Autodesk Fusion 360 part; units mm, degrees
(part 3 of 4)
  measures "d44" distance of L104.start L104.end
  measures "d45" distance of L104.start L106.end
  measures "d46" distance of L108.start L108.end
  measures "d47" distance of L108.start L110.end
  measures "d48" distance of L112.start L112.end
  measures "d49" distance of L112.start L114.end
  measures "d50" distance of L116.start L116.end
  measures "d51" distance of L116.start L118.end
  measures "d52" distance of L120.start L120.end
  measures "d53" distance of L120.start L122.end
  measures "d54" distance of L124.start L124.end
  measures "d55" distance of L124.start L126.end
  measures "d56" distance of L128.start L128.end
  measures "d57" distance of L128.start L130.end
  measures "d58" distance of L132.start L132.end
  measures "d59" distance of L132.start L134.end
  measures "d60" distance of L136.start L136.end
  measures "d61" distance of L136.start L138.end
  measures "d62" distance of L140.start L140.end
  measures "d63" distance of L140.start L142.end
  measures "d64" distance of L144.start L144.end
  measures "d65" distance of L144.start L146.end
  measures "d66" distance of L18.end L148.end
  measures "d67" distance of L18.end L150.end
  measures "d68" distance of L26.end L152.end
  measures "d69" distance of L26.end L154.end
  measures "d70" distance of L34.end L156.end
  measures "d71" distance of L34.end L158.end
  measures "d72" distance of L160.start L160.end
  measures "d73" distance of L160.start L162.end
  measures "d74" distance of L164.start L164.end
  measures "d75" distance of L164.start L166.end
  measures "d76" distance of L168.start L168.end
  measures "d77" distance of L168.start L170.end
  measures "d78" distance of L172.start L172.end
  measures "d79" distance of L172.start L174.end
  measures "d80" distance of L176.start L176.end
  measures "d81" distance of L176.start L178.end
  measures "d82" distance of L180.start L180.end
  measures "d83" distance of L180.start L182.end
  measures "d84" distance of L184.start L184.end
  measures "d85" distance of L184.start L186.end
  measures "d86" distance of L188.start L188.end
  measures "d87" distance of L188.start L190.end
  measures "d88" distance of L192.start L192.end
  measures "d89" distance of L192.start L194.end
  measures "d90" distance of L196.start L196.end
  measures "d91" distance of L196.start L198.end
  measures "d92" distance of L200.start L200.end
  measures "d93" distance of L200.start L202.end
  measures "d94" distance of L86.end L204.end
  measures "d95" distance of L86.end L206.end
  measures "d96" distance of L94.end L208.end
  measures "d97" distance of L94.end L210.end
  measures "d98" distance of L212.start L212.end
  measures "d99" distance of L212.start L214.end
  measures "d100" distance of L78.end L216.end
  measures "d101" distance of L78.end L218.end
  measures "d102" distance of L70.end L220.end
  measures "d103" distance of L70.end L222.end
  measures "d104" distance of L42.end L224.end
  measures "d105" distance of L42.end L226.end
  measures "d106" distance of L50.end L228.end
  measures "d107" distance of L50.end L230.end
  measures "d108" distance of L58.end L232.end
  measures "d109" distance of L58.end L234.end
  measures "d110" distance of L0.end L236.end
  measures "d111" distance of L0.end L238.end
  measures "d112" diameter of A0
  measures "d113" diameter of A1
  measures "d114" diameter of A2
  measures "d115" diameter of A3
  measures "d116" diameter of A4
  measures "d117" diameter of A5
  measures "d118" diameter of A6
  measures "d119" diameter of A7
  measures "d120" diameter of A8
  measures "d121" diameter of A9
  measures "d122" diameter of A10
  measures "d123" diameter of A11
  measures "d124" diameter of A12
  measures "d125" diameter of A13
  measures "d126" diameter of A14
  measures "d127" diameter of A15
  measures "d128" diameter of A16
  measures "d129" diameter of A17
  measures "d130" diameter of A18
  measures "d131" diameter of A19
  measures "d132" diameter of A20
  measures "d133" diameter of A21
  measures "d134" diameter of A22
  measures "d135" diameter of A23
  measures "d136" diameter of A24
  measures "d137" diameter of A25
  measures "d138" diameter of A26
  measures "d139" diameter of A27
  measures "d140" diameter of A28
  measures "d141" diameter of A29
  measures "d142" diameter of A30
  measures "d143" diameter of A31
  measures "d144" diameter of A32
  measures "d146" diameter of A33
  measures "d149" distance of L12 A21.centre
  measures "d150" distance of A21.centre A23.centre
  measures "d151" distance of P2 A23.centre
  measures "d152" distance of P3 P2
  measures "d154" distance of L148 A0.centre
  measures "d155" distance of L7 A21.centre
  measures "d156" distance of A21.centre A22.centre
  measures "d157" distance of A22.centre A25.centre
  measures "d158" distance of A25.centre A27.centre
  measures "d159" distance of A27.centre A29.centre
  measures "d160" distance of A29.centre A31.centre
  measures "d164" distance of A32.centre A33.centre
  measures "d167" distance of A14.centre A15.centre
  measures "d168" distance of L240.start L240.end
  measures "d169" distance of L241.start L241.end
  measures "d170" distance of A10.centre A17.centre
  measures "d171" distance of L0 A0.centre
  measures "d172" horizontal distance of L238.end A6.centre
  measures "d173" distance of L95 A7.centre
  measures "d174" distance of L87 A14.centre
  measures "d175" distance of L79 A33.centre
  measures "d177" diameter of A34
extrude "Extrude4" cut sketch "Sketch3" against normal blind 50 contours L217 A33 L247 | L217 A33 L247 | L205 A14 L247 | L205 A14 L247 | L209 A7 L247 | L209 A7 L247 | A21 L242 | A21 L242 | A23 L242 L243 | A23 L242 L243 | A23 L242 L243 | A23 L242 L243 | A20 L242 L244 | A20 L242 L244 | A20 L242 L244 | A20 L242 L244 | A13 L242 L245 | A13 L242 L245 | A13 L242 L245 | A13 L242 L245 | A0 L240 L246 | A0 L240 L242 | A0 L240 L242 L246 | L154 A1 L246 | L154 A1 L246 | L158 A2 L246 | L158 A2 L246 | L201 A15 | L201 A15 | L226 A3 L246 | L226 A3 L246 | L230 A4 L246 | L230 A4 L246 | L234 A5 L246 | L234 A5 L246 | L237 A6 L246 | L237 L238 A6 L246 | L238 A6 L246 L247 | A6 L246 L247 | A8 | A9 | A10 | A11 | A12 | A16 | A17 | A18 | A19 | A22 | A24 | A25 | A26 | A27 | A28 | A29 | A30 | A31 | A32
extrude "Extrude3" cut sketch "Sketch3" against normal blind 50 contours L221 L247 A34 | L221 L247 A34 | L217 A33 L247 | L217 A33 L247 | L205 A14 L247 | L205 A14 L247 | L209 A7 L247 | L209 A7 L247 | A21 L242 | A21 L242 | A23 L242 L243 | A23 L242 L243 | A23 L242 L243 | A23 L242 L243 | A20 L242 L244 | A20 L242 L244 | A20 L242 L244 | A20 L242 L244 | A13 L242 L245 | A13 L242 L245 | A13 L242 L245 | A13 L242 L245 | A0 L240 L246 | A0 L240 L242 | A0 L240 L242 L246 | L154 A1 L246 | L154 A1 L246 | L158 A2 L246 | L158 A2 L246 | L201 A15 | L201 A15 | L226 A3 L246 | L226 A3 L246 | L230 A4 L246 | L230 A4 L246 | L234 A5 L246 | L234 A5 L246 | L237 A6 L246 | L237 L238 A6 L246 | L238 A6 L246 L247 | A6 L246 L247 | A8 | A9 | A10 | A11 | A12 | A16 | A17 | A18 | A19 | A22 | A24 | A25 | A26 | A27 | A28 | A29 | A30 | A31 | A32

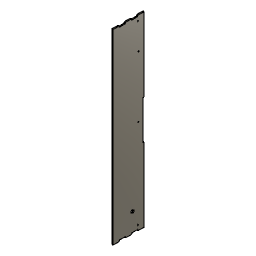
design "C2. Bordes Laterales.Salida fuente.v3"
Autodesk Fusion 360 part; units mm, degrees
ref_plane "WorkPlane1" through (0, 3, 0) normal (0, 1, 0) x (0, 0, 1)
sketch "Sketch1" plane through (0, 3, 0) normal (0, 1, 0) x (1, 0, 0)
  line L0 (340.5, 241.5) -> (-340.5, 241.5) construction
  line L1 (-340.5, 241.5) -> (-340.5, -241.5) construction
  line L2 (-340.5, -241.5) -> (340.5, -241.5) construction
  line L3 (340.5, -241.5) -> (340.5, 241.5) construction
  line L4 (340.5, 241.5) -> (-340.5, -241.5) construction
  line L5 (-340.5, 241.5) -> (340.5, -241.5) construction
  line L6 (-340.5, 241.5) -> (-337.5, 241.5)
  line L7 (-337.5, 241.5) -> (-337.5, -241.5)
  line L8 (-337.5, -241.5) -> (-340.5, -241.5)
  line L9 (-340.5, -241.5) -> (-340.5, 241.5)
  dimension "d2" = 681
  dimension "d3" = 483
  dimension "d4" = 3
  constraint horizontal L0
  constraint perpendicular L0 L1
  constraint parallel L0 L2
  constraint parallel L1 L3
  constraint coincident L4 origin
  constraint coincident L5 origin
  constraint horizontal L6
  constraint vertical L7
  constraint horizontal L8
  constraint vertical L9
  measures "d2" distance of L1.end L2.end
  measures "d3" distance of L0.end L1.end
  measures "d4" distance of L0.end L6.end
extrude "Extrude1" add sketch "Sketch1" along normal blind 80
ref_plane "WorkPlane2" through (-340.5, 43, 0) normal (-1, 0, 0) x (0, 0, 1)
sketch "Sketch2" plane through (-340.5, 42, 0) normal (-1, 0, 0) x (0, 1, 0)
  line L0 (-39, 241.5) -> (-39, -241.5)
  line L1 (-39, -241.5) -> (41, -241.5)
  line L2 (41, -241.5) -> (41, 241.5)
  line L3 (41, 241.5) -> (-39, 241.5)
  line L4 (0, 0) -> (0, -50) construction
  line L5 (0, 0) -> (0, 50) construction
  line L6 (41, 50) -> (38, 50)
  line L7 (38, 50) -> (38, -50)
  line L8 (38, -50) -> (41, -50)
  line L9 (41, -50) -> (41, 50)
  line L10 (-39, 241.5) -> (-23, 241.5)
  line L11 (-23, 241.5) -> (-23, 244.5)
  line L12 (-23, 244.5) -> (-39, 244.5)
  line L13 (-39, 244.5) -> (-39, 241.5)
  line L14 (-23, 241.5) -> (-7, 241.5)
  line L15 (-7, 241.5) -> (-7, 238.5)
  line L16 (-7, 238.5) -> (-23, 238.5)
  line L17 (-23, 238.5) -> (-23, 241.5)
  line L18 (-7, 241.5) -> (9, 241.5)
  line L19 (9, 241.5) -> (9, 244.5)
  line L20 (9, 244.5) -> (-7, 244.5)
  line L21 (-7, 244.5) -> (-7, 241.5)
  line L22 (9, 241.5) -> (25, 241.5)
  line L23 (25, 241.5) -> (25, 238.5)
  line L24 (25, 238.5) -> (9, 238.5)
  line L25 (9, 238.5) -> (9, 241.5)
  line L26 (-39, -241.5) -> (-23, -241.5)
  line L27 (-23, -241.5) -> (-23, -244.5)
  line L28 (-23, -244.5) -> (-39, -244.5)
  line L29 (-39, -244.5) -> (-39, -241.5)
  line L30 (-23, -241.5) -> (-7, -241.5)
  line L31 (-7, -241.5) -> (-7, -238.5)
  line L32 (-7, -238.5) -> (-23, -238.5)
  line L33 (-23, -238.5) -> (-23, -241.5)
  line L34 (-7, -241.5) -> (9, -241.5)
  line L35 (9, -241.5) -> (9, -244.5)
  line L36 (9, -244.5) -> (-7, -244.5)
  line L37 (-7, -244.5) -> (-7, -241.5)
  line L38 (9, -241.5) -> (25, -241.5)
  line L39 (25, -241.5) -> (25, -238.5)
  line L40 (25, -238.5) -> (9, -238.5)
  line L41 (9, -238.5) -> (9, -241.5)
  line L42 (25, -241.5) -> (40, -241.5)
  line L43 (25, -241.5) -> (41, -241.5)
  line L44 (41, -241.5) -> (41, -244.5)
  line L45 (41, -244.5) -> (25, -244.5)
  line L46 (25, -244.5) -> (25, -241.5)
  line L47 (25, 241.5) -> (41, 241.5)
  line L48 (41, 241.5) -> (41, 244.5)
  line L49 (41, 244.5) -> (25, 244.5)
  line L50 (25, 244.5) -> (25, 241.5)
  dimension "d8" = 50
  dimension "d9" = 50
  dimension "d10" = 3
  dimension "d11" = 16
  dimension "d12" = 3
  dimension "d13" = 16
  dimension "d14" = 3
  dimension "d15" = 16
  dimension "d16" = 3
  dimension "d17" = 16
  dimension "d18" = 3
  dimension "d20" = 16
  dimension "d21" = 3
  dimension "d22" = 16
  dimension "d23" = 3
  dimension "d24" = 16
  dimension "d25" = 3
  dimension "d26" = 16
  dimension "d27" = 3
  dimension "d31" = 3
  dimension "d32" = 3
  constraint coincident L4.start L5.start
  constraint parallel L0 L4
  constraint vertical L5
  constraint horizontal L6
  constraint vertical L7
  constraint horizontal L8
  constraint vertical L9
  constraint coincident L2 L6.start
  constraint horizontal L10
  constraint vertical L11
  constraint horizontal L12
  constraint vertical L13
  constraint coincident L0.start L3.end
  constraint horizontal L14
  constraint vertical L15
  constraint horizontal L16
  constraint vertical L17
  constraint horizontal L18
  constraint vertical L19
  constraint horizontal L20
  constraint vertical L21
  constraint horizontal L22
  constraint vertical L23
  constraint horizontal L24
  constraint vertical L25
  constraint horizontal L26
  constraint vertical L27
  constraint horizontal L28
  constraint vertical L29
  constraint coincident L0.end L1.start
  constraint horizontal L30
  constraint vertical L31
  constraint horizontal L32
  constraint vertical L33
  constraint horizontal L34
  constraint vertical L35
  constraint horizontal L36
  constraint vertical L37
  constraint horizontal L38
  constraint vertical L39
  constraint horizontal L40
  constraint vertical L41
  constraint horizontal L42
  constraint horizontal L43
  constraint vertical L44
  constraint horizontal L45
  constraint vertical L46
  constraint horizontal L47
  constraint vertical L48
  constraint horizontal L49
  constraint vertical L50
  measures "d8" distance of L4.start L4.end
  measures "d9" distance of L4.start L5.end
  measures "d10" distance of L6.start L6.end
  measures "d11" distance of L0.start L10.end
  measures "d12" distance of L0.start L12.end
  measures "d13" distance of L10.end L14.end
  measures "d14" distance of L10.end L16.end
  measures "d15" distance of L14.end L18.end
  measures "d16" distance of L14.end L20.end
  measures "d17" distance of L18.end L22.end
  measures "d18" distance of L18.end L24.end
  measures "d20" distance of L0.end L26.end
  measures "d21" distance of L0.end L28.end
  measures "d22" distance of L26.end L30.end
  measures "d23" distance of L26.end L32.end
  measures "d24" distance of L30.end L34.end
  measures "d25" distance of L30.end L36.end
  measures "d26" distance of L34.end L38.end
  measures "d27" distance of L34.end L40.end
  measures "d31" distance of L38.end L45.end
  measures "d32" distance of L22.end L49.end
extrude "Extrude2" cut sketch "Sketch2" against normal blind 25 contours L3 L14 L15 L16 L17 | L1 L30 L31 L32 L33 | L3 L22 L23 L24 L25 | L1 L38 L39 L40 L41 | L2 L6 L7 L8 L9
ref_plane "WorkPlane3" through (-337.5, 43, 0) normal (1, 0, 0) x (0, 0, -1)
sketch "Sketch3" plane through (-337.5, 43, 0) normal (1, 0, 0) x (0, 1, 0)
  line L0 (37, 50) -> (40, 50)
  line L1 (40, 50) -> (40, 241.5)
  line L2 (40, 241.5) -> (24, 241.5)
  line L3 (24, 241.5) -> (24, 238.5)
  line L4 (24, 238.5) -> (8, 238.5)
  line L5 (8, 238.5) -> (8, 241.5)
  line L6 (8, 241.5) -> (-8, 241.5)
  line L7 (-8, 241.5) -> (-8, 238.5)
  line L8 (-8, 238.5) -> (-24, 238.5)
  line L9 (-24, 238.5) -> (-24, 241.5)
  line L10 (-24, 241.5) -> (-40, 241.5)
  line L11 (-40, 241.5) -> (-40, -241.5)
  line L12 (-40, -241.5) -> (-24, -241.5)
  line L13 (-24, -241.5) -> (-24, -238.5)
  line L14 (-24, -238.5) -> (-8, -238.5)
  line L15 (-8, -238.5) -> (-8, -241.5)
  line L16 (-8, -241.5) -> (8, -241.5)
  line L17 (8, -241.5) -> (8, -238.5)
  line L18 (8, -238.5) -> (24, -238.5)
  line L19 (24, -238.5) -> (24, -241.5)
  line L20 (24, -241.5) -> (40, -241.5)
  line L21 (40, -241.5) -> (40, -50)
  line L22 (40, -50) -> (37, -50)
  line L23 (37, -50) -> (37, 50)
ref_plane "WorkPlane4" through (-337.5, 43, 0) normal (1, 0, 0) x (0, 0, -1)
sketch "Sketch4" plane through (-337.5, 43, 0) normal (1, 0, 0) x (0, 1, 0)
  line L0 (37, -50) -> (37, 50)
  line L1 (37, 10) -> (19, 10)
  line L2 (19, 10) -> (19, -10)
  line L3 (19, -10) -> (37, -10)
  line L4 (37, -10) -> (37, 10)
  line L5 (37, 10) -> (19, -10) construction
  line L6 (19, 10) -> (37, -10) construction
  circle A0 centre (25, 2) radius 1.5
  circle A1 centre (10, -191.5) radius 4
  line L7 (37, 50) -> (37, 260) construction
  circle A2 centre (24, 228.5) radius 1.5
  line L8 (19, 238.5) -> (19, 218.5)
  line L9 (19, 218.5) -> (37, 218.5)
  line L10 (37, 218.5) -> (37, 238.5)
  line L11 (37, 238.5) -> (19, 238.5)
  line L12 (0, 0) -> (6.2879, 0)
  circle A3 centre (24, -228.5) radius 1.5
  line L13 (19, -218.5) -> (37, -218.5)
  line L14 (37, -218.5) -> (37, -238.5)
  line L15 (37, -238.5) -> (19, -238.5)
  line L16 (19, -238.5) -> (19, -218.5)
  line L17 (40, 241.5) -> (45, 241.5)
  line L18 (45, 241.5) -> (45, 141.5)
  line L19 (37, 161.5) -> (19, 161.5)
  line L20 (19, 161.5) -> (19, 141.5)
  line L21 (19, 141.5) -> (37, 141.5)
  line L22 (37, 141.5) -> (37, 161.5)
  circle A4 centre (26, 159.346) radius 1.5
  line L23 (37, 238.5) -> (42, 238.5)
  line L24 (42, 238.5) -> (42, 161.5)
  line L25 (40, 241.5) -> (40, 50)
  line L26 (24, 241.5) -> (40, 241.5)
  line L27 (28, 241.5) -> (28, 228.5)
  line L28 (24, -241.5) -> (40, -241.5)
  line L29 (40, -50) -> (40, -241.5)
  line L30 (87.333, 241.5) -> (87.333, 159.346)
  line L31 (87.333, 159.346) -> (-5, 159.346)
  point P0 (-0.5, -125.5)
  point P1 (28, 0)
  point P2 (37, 238.5)
  point P3 (37, -238.5)
  point P4 (40, 241.5)
  point P5 (26, 159.346)
  dimension "d47" = 20
  dimension "d53" = 3
  dimension "d54" = 18
  dimension "d61" = 8
  dimension "d64" = 3
  dimension "d65" = 18
  dimension "d66" = 100
  dimension "d67" = 3
  dimension "d68" = 18
  dimension "d69" = 77
  dimension "d70" = 13
  dimension "d71" = 16
  dimension "d72" = 13
  dimension "d73" = 12
  dimension "d74" = 14
  dimension "d75" = 12
  dimension "d76" = 16
  dimension "d77" = 82.154
  dimension "d78" = 82.154
  constraint horizontal L1
  constraint perpendicular L1 L2
  constraint parallel L1 L3
  constraint parallel L2 L4
  constraint coincident L5 P1
  constraint coincident L6 P1
  constraint horizontal L11
  constraint vertical L8
  constraint horizontal L9
  constraint vertical L10
  constraint coincident L12.start origin
  constraint horizontal L12
  constraint symmetric P2 L12 P3
  constraint symmetric L8.end L12 L13.start
  constraint symmetric L8.start L12 L15.end
  constraint symmetric L9.end L12 L13.end
  constraint symmetric A2 L12 A3
  constraint coincident P4 L17.start
  constraint perpendicular L7 L17
  constraint perpendicular L11 L18
  constraint horizontal L19
  constraint vertical L20
  constraint horizontal L21
  constraint vertical L22
  constraint coincident P2 L10.end
  constraint perpendicular L10 L23
  constraint perpendicular L19 L24
  constraint coincident L26 L27.start
  constraint perpendicular L26 L27
  constraint perpendicular L17 L30
  constraint perpendicular L22 L31
  constraint coincident L31 P5
  measures "d47" distance of L1.end L2.end
  measures "d53" diameter of A0
  measures "d54" distance of L1.start L1.end
  measures "d61" diameter of A1
  measures "d64" diameter of A2
  measures "d65" distance of P2 L8.start
  measures "d66" distance of L17.end L18.end
  measures "d67" diameter of A4
  measures "d68" distance of L19.end L19.start
  measures "d69" distance of L23.end L24.end
  measures "d70" distance of L27.start L27.end
  measures "d71" distance of A3.centre L29
  measures "d72" distance of A3.centre L28
  measures "d73" distance of L4 A0.centre
  measures "d74" distance of P5 L25
  measures "d75" distance of L25 L27.end
  measures "d76" distance of A2.centre L25
  measures "d77" distance of L30.start L30.end
  measures "d78" distance of L30.start L30.end
extrude "Extrude3" cut sketch "Sketch4" against normal blind 20 contours A0 | A1 | A2 | A3 | A4 L31 | A4 L31

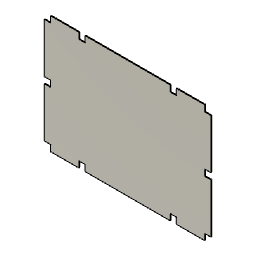
design "D.Pantalla cartnegro.v3"
Autodesk Fusion 360 part; units mm, degrees
ref_plane "WorkPlane1" through (0, 22, 0) normal (0, 1, 0) x (0, 0, 1)
sketch "Sketch1" plane through (0, 22, 0) normal (0, 1, 0) x (1, 0, 0)
  line L0 (337.5, -238.5) -> (-337.5, -238.5)
  line L1 (-337.5, -238.5) -> (-337.5, 238.5)
  line L2 (-337.5, 238.5) -> (337.5, 238.5)
  line L3 (337.5, 238.5) -> (337.5, -238.5)
  line L4 (337.5, -238.5) -> (-337.5, 238.5) construction
  line L5 (-337.5, -238.5) -> (337.5, 238.5) construction
  dimension "d2" = 675
  dimension "d3" = 477
  constraint horizontal L0
  constraint perpendicular L0 L1
  constraint parallel L0 L2
  constraint parallel L1 L3
  constraint coincident L4 origin
  constraint coincident L5 origin
  measures "d2" distance of L1.end L2.end
  measures "d3" distance of L0.end L1.end
extrude "Extrude1" add sketch "Sketch1" along normal blind 3
ref_plane "WorkPlane2" through (0, 22, 0) normal (0, -1, 0) x (-1, 0, 0)
sketch "Sketch2" plane through (0, 22, 0) normal (0, -1, 0) x (1, 0, 0)
  line L0 (-337.5, -238.5) -> (337.5, -238.5)
  line L1 (337.5, -238.5) -> (337.5, 238.5)
  line L2 (337.5, 238.5) -> (-337.5, 238.5)
  line L3 (-337.5, 238.5) -> (-337.5, -238.5)
  line L4 (337.5, 238.5) -> (312.5, 238.5)
  line L5 (312.5, 238.5) -> (312.5, 213.5)
  line L6 (312.5, 213.5) -> (337.5, 213.5)
  line L7 (337.5, 213.5) -> (337.5, 238.5)
  line L8 (-337.5, 238.5) -> (-312.5, 238.5)
  line L9 (-312.5, 238.5) -> (-312.5, 213.5)
  line L10 (-312.5, 213.5) -> (-337.5, 213.5)
  line L11 (-337.5, 213.5) -> (-337.5, 238.5)
  line L12 (-337.5, -238.5) -> (-312.5, -238.5)
  line L13 (-312.5, -238.5) -> (-312.5, -213.5)
  line L14 (-312.5, -213.5) -> (-337.5, -213.5)
  line L15 (-337.5, -213.5) -> (-337.5, -238.5)
  line L16 (337.5, -238.5) -> (312.5, -238.5)
  line L17 (312.5, -238.5) -> (312.5, -213.5)
  line L18 (312.5, -213.5) -> (337.5, -213.5)
  line L19 (337.5, -213.5) -> (337.5, -238.5)
  line L20 (337.5, 12.5) -> (312.5, 12.5)
  line L21 (312.5, 12.5) -> (312.5, -12.5)
  line L22 (312.5, -12.5) -> (337.5, -12.5)
  line L23 (337.5, -12.5) -> (337.5, 12.5)
  line L24 (337.5, 12.5) -> (312.5, -12.5) construction
  line L25 (312.5, 12.5) -> (337.5, -12.5) construction
  line L26 (-337.5, 12.5) -> (-337.5, -12.5)
  line L27 (-312.5, -12.5) -> (-312.5, 12.5)
  line L28 (-312.5, -238.5) -> (-312.5, 238.5)
  line L29 (-337.5, -12.5) -> (-312.5, -12.5)
  line L30 (-337.5, 12.5) -> (-312.5, -12.5) construction
  line L31 (-312.5, 12.5) -> (-337.5, -12.5) construction
  line L32 (-312.5, 12.5) -> (-337.5, 12.5)
  line L33 (-337.5, 262.49) -> (-197.5, 262.49)
  line L34 (-337.5, -260.2374) -> (-197.5, -260.2374)
  line L35 (337.5, 281.2113) -> (197.5, 281.2113)
  line L36 (-197.5, 238.5) -> (-172.5, 238.5)
  line L37 (-172.5, 238.5) -> (-172.5, 213.5)
  line L38 (-172.5, 213.5) -> (-197.5, 213.5)
  line L39 (-197.5, 213.5) -> (-197.5, 238.5)
  line L40 (197.5, 238.5) -> (172.5, 238.5)
  line L41 (172.5, 238.5) -> (172.5, 213.5)
  line L42 (172.5, 213.5) -> (197.5, 213.5)
  line L43 (197.5, 213.5) -> (197.5, 238.5)
  line L44 (337.5, -262.9157) -> (197.5, -262.9157)
  line L45 (197.5, -238.5) -> (172.5, -238.5)
  line L46 (172.5, -238.5) -> (172.5, -213.5)
  line L47 (172.5, -213.5) -> (197.5, -213.5)
  line L48 (197.5, -213.5) -> (197.5, -238.5)
  line L49 (-197.5, -238.5) -> (-172.5, -238.5)
  line L50 (-172.5, -238.5) -> (-172.5, -213.5)
  line L51 (-172.5, -213.5) -> (-197.5, -213.5)
  line L52 (-197.5, -213.5) -> (-197.5, -238.5)
  point P0 (337.5, 0)
  point P1 (325, 0)
  point P2 (-312.5, 0)
  point P3 (-325, 0)
  dimension "d7" = 25
  dimension "d8" = 25
  dimension "d9" = 25
  dimension "d10" = 25
  dimension "d11" = 25
  dimension "d12" = 25
  dimension "d13" = 25
  dimension "d14" = 25
  dimension "d17" = 140
  dimension "d18" = 140
  dimension "d19" = 140
  dimension "d20" = 25
  dimension "d21" = 25
  dimension "d22" = 25
  dimension "d23" = 25
  dimension "d24" = 140
  dimension "d25" = 25
  dimension "d26" = 25
  dimension "d27" = 25
  dimension "d28" = 25
  constraint horizontal L4
  constraint vertical L5
  constraint horizontal L6
  constraint vertical L7
  constraint coincident L1.end L2.start
  constraint horizontal L8
  constraint vertical L9
  constraint horizontal L10
  constraint vertical L11
  constraint coincident L2.end L3.start
  constraint horizontal L12
  constraint vertical L13
  constraint horizontal L14
  constraint vertical L15
  constraint coincident L0.start L3.end
  constraint horizontal L16
  constraint vertical L17
  constraint horizontal L18
  constraint vertical L19
  constraint coincident L0.end L1.start
  constraint horizontal L20
  constraint perpendicular L20 L21
  constraint parallel L20 L22
  constraint parallel L21 L23
  constraint coincident L24 P1
  constraint coincident L25 P1
  constraint horizontal L32
  constraint perpendicular L26 L32
  constraint parallel L29 L32
  constraint parallel L26 L27
  constraint coincident P3 L31
  constraint coincident P3 L30
  constraint perpendicular L3 L33
  constraint horizontal L34
  constraint perpendicular L7 L35
  constraint horizontal L36
  constraint vertical L37
  constraint horizontal L38
  constraint vertical L39
  constraint coincident L2 L36.start
  constraint horizontal L40
  constraint vertical L41
  constraint horizontal L42
  constraint vertical L43
  constraint coincident L2 L40.start
  constraint perpendicular L1 L44
  constraint horizontal L45
  constraint vertical L46
  constraint horizontal L47
  constraint vertical L48
  constraint coincident L0 L45.start
  constraint horizontal L49
  constraint vertical L50
  constraint horizontal L51
  constraint vertical L52
  constraint coincident L0 L49.start
  measures "d7" distance of L1.end L4.end
  measures "d8" distance of L1.end L6.end
  measures "d9" distance of L2.end L8.end
  measures "d10" distance of L2.end L10.end
  measures "d11" distance of L0.start L12.end
  measures "d12" distance of L0.start L14.end
  measures "d13" distance of L0.end L16.end
  measures "d14" distance of L0.end L18.end
  measures "d17" distance of L33.start L33.end
  measures "d18" distance of L34.start L34.end
  measures "d19" distance of L35.start L35.end
  measures "d20" distance of L36.start L36.end
  measures "d21" distance of L36.start L38.end
  measures "d22" distance of L40.start L40.end
  measures "d23" distance of L40.start L42.end
  measures "d24" distance of L44.start L44.end
  measures "d25" distance of L45.start L45.end
  measures "d26" distance of L45.start L47.end
  measures "d27" distance of L49.start L49.end
  measures "d28" distance of L49.start L51.end
extrude "Extrude2" cut sketch "Sketch2" against normal blind 150 contours L0 L3 L12 L13 L14 L15 L28 | L0 L49 L50 L51 L52 | L3 L26 L27 L28 L29 L32 | L0 L45 L46 L47 L48 | L2 L3 L8 L9 L10 L11 L28 | L0 L1 L16 L17 L18 L19 | L2 L36 L37 L38 L39 | L1 L20 L21 L22 L23 | L2 L40 L41 L42 L43 | L1 L2 L4 L5 L6 L7
ref_plane "WorkPlane3" through (0, 22, 0) normal (0, -1, 0) x (-1, 0, 0)
sketch "Sketch3" plane through (0, 22, 0) normal (0, -1, 0) x (1, 0, 0)
  line L0 (82.5, 1.5) -> (82.5, 16.5)
  line L1 (163.5, 16.5) -> (178.5, 16.5)
  line L2 (178.5, 241.5) -> (181.5, 241.5) construction
  circle A0 centre (171, 90) radius 1.5
  line L3 (178.5, 163.5) -> (100.5, 163.5)
  line L4 (178.5, 82.5) -> (163.5, 82.5)
  line L5 (97.5, 241.5) -> (97.5, 163.5) construction
  line L6 (181.5, 163.5) -> (181.5, 241.5) construction
  line L7 (97.5, 82.5) -> (82.5, 82.5)
  line L8 (-340.5, -82.5) -> (340.5, -82.5) construction
  line L9 (19.5, 241.5) -> (97.5, 241.5) construction
  line L10 (97.5, 241.5) -> (100.5, 241.5) construction
  line L11 (340.5, -1.5) -> (-340.5, -1.5) construction
  line L12 (82.5, 82.5) -> (82.5, 97.5)
  line L13 (97.5, 97.5) -> (97.5, 82.5)
  line L14 (340.5, 82.5) -> (340.5, 160.5)
  line L15 (259.5, 241.5) -> (259.5, 163.5) construction
  line L16 (178.5, 241.5) -> (178.5, 163.5) construction
  circle A1 centre (90, 90) radius 1.5
  line L17 (244.5, 82.5) -> (244.5, 97.5)
  line L18 (244.5, 16.5) -> (259.5, 16.5)
  line L19 (340.5, 97.5) -> (340.5, 82.5)
  circle A2 centre (171, 9) radius 1.5
  line L20 (82.5, 97.5) -> (97.5, 97.5)
  line L21 (97.5, 16.5) -> (97.5, 1.5)
  line L22 (100.5, 241.5) -> (178.5, 241.5) construction
  line L23 (340.5, 79.5) -> (340.5, 82.5)
  line L24 (340.5, 163.5) -> (262.5, 163.5)
  line L25 (100.5, 163.5) -> (100.5, 241.5) construction
  line L26 (178.5, 16.5) -> (178.5, 1.5)
  line L27 (82.5, 16.5) -> (97.5, 16.5)
  line L28 (97.5, 163.5) -> (19.5, 163.5)
  line L29 (163.5, 97.5) -> (178.5, 97.5)
  line L30 (178.5, 97.5) -> (178.5, 82.5)
  circle A3 centre (90, 9) radius 1.5
  line L31 (163.5, 82.5) -> (163.5, 97.5)
  line L32 (97.5, 1.5) -> (82.5, 1.5)
  line L33 (178.5, 1.5) -> (163.5, 1.5)
  line L34 (163.5, 1.5) -> (163.5, 16.5)
  line L35 (163.5, -64.5) -> (178.5, -64.5)
  line L36 (97.5, -79.5) -> (82.5, -79.5)
  circle A4 centre (90, -234) radius 1.5
  line L37 (97.5, -241.5) -> (82.5, -241.5)
  line L38 (340.5, 79.5) -> (-340.5, 79.5) construction
  line L39 (82.5, -79.5) -> (82.5, -64.5)
  line L40 (-340.5, -163.5) -> (340.5, -163.5) construction
  line L41 (163.5, -226.5) -> (178.5, -226.5)
  line L42 (-340.5, 82.5) -> (340.5, 82.5) construction
  line L43 (340.5, 163.5) -> (-340.5, 163.5) construction
  line L44 (97.5, -64.5) -> (97.5, -79.5)
  line L45 (82.5, -241.5) -> (82.5, -226.5)
  line L46 (163.5, -241.5) -> (163.5, -226.5)
  line L47 (163.5, -145.5) -> (178.5, -145.5)
  line L48 (-340.5, -1.5) -> (340.5, -1.5) construction
  line L49 (178.5, -226.5) -> (178.5, -241.5)
  line L50 (82.5, -64.5) -> (97.5, -64.5)
  line L51 (340.5, 241.5) -> (-340.5, 241.5) construction
  line L52 (163.5, -79.5) -> (163.5, -64.5)
  line L53 (97.5, -226.5) -> (97.5, -241.5)
  circle A5 centre (171, -153) radius 1.5
  line L54 (340.5, -1.5) -> (340.5, 1.5)
  circle A6 centre (252, 9) radius 1.5
  line L55 (325.5, 1.5) -> (325.5, 16.5)
  line L56 (97.5, -160.5) -> (82.5, -160.5)
  line L57 (259.5, 82.5) -> (244.5, 82.5)
  line L58 (340.5, 82.5) -> (325.5, 82.5)
  line L59 (340.5, -145.5) -> (340.5, -160.5)
  circle A7 centre (333, -72) radius 1.5
  line L60 (244.5, -160.5) -> (244.5, -145.5)
  line L61 (340.5, -79.5) -> (340.5, -1.5)
  line L62 (16.5, -226.5) -> (16.5, -241.5)
  line L63 (16.5, 16.5) -> (16.5, 1.5)
  circle A8 centre (252, -153) radius 1.5
  line L64 (244.5, -145.5) -> (259.5, -145.5)
  line L65 (340.5, -160.5) -> (325.5, -160.5)
  line L66 (325.5, -145.5) -> (340.5, -145.5)
  line L67 (244.5, -241.5) -> (244.5, -226.5)
  line L68 (325.5, -160.5) -> (325.5, -145.5)
  line L69 (19.5, 163.5) -> (19.5, 241.5) construction
  circle A9 centre (333, -153) radius 1.5
  line L70 (259.5, -226.5) -> (259.5, -241.5)
  line L71 (259.5, -79.5) -> (244.5, -79.5)
  line L72 (325.5, -241.5) -> (325.5, -226.5)
  line L73 (340.5, -241.5) -> (325.5, -241.5)
  line L74 (340.5, -163.5) -> (340.5, -160.5)
  line L75 (259.5, -241.5) -> (244.5, -241.5)
  line L76 (-223.5, 241.5) -> (-223.5, -241.5) construction
  line L77 (340.5, -64.5) -> (340.5, -79.5)
  line L78 (-142.5, 241.5) -> (-64.5, 241.5) construction
  line L79 (-61.5, 241.5) -> (16.5, 241.5) construction
  line L80 (-226.5, 241.5) -> (-226.5, -241.5) construction
  circle A10 centre (252, -72) radius 1.5
  line L81 (340.5, -79.5) -> (325.5, -79.5)
  line L82 (-64.5, 82.5) -> (-79.5, 82.5)
  line L83 (340.5, -82.5) -> (340.5, -79.5)
  line L84 (1.5, 82.5) -> (1.5, 97.5)
  circle A11 centre (252, -234) radius 1.5
  line L85 (16.5, -241.5) -> (16.5, 241.5) construction
  line L86 (262.5, -241.5) -> (259.5, -241.5)
  line L87 (-79.5, 16.5) -> (-64.5, 16.5)
  line L88 (244.5, -64.5) -> (259.5, -64.5)
  line L89 (-340.5, 241.5) -> (-340.5, -241.5) construction
  line L90 (178.5, -64.5) -> (178.5, -79.5)
  circle A12 centre (90, -153) radius 1.5
  line L91 (82.5, -145.5) -> (97.5, -145.5)
  line L92 (97.5, -145.5) -> (97.5, -160.5)
  circle A13 centre (171, -234) radius 1.5
  line L93 (178.5, -145.5) -> (178.5, -160.5)
  line L94 (178.5, -79.5) -> (163.5, -79.5)
  line L95 (178.5, -160.5) -> (163.5, -160.5)
  line L96 (181.5, -241.5) -> (178.5, -241.5)
  line L97 (163.5, -160.5) -> (163.5, -145.5)
  circle A14 centre (90, -72) radius 1.5
  line L98 (100.5, -241.5) -> (97.5, -241.5)
  line L99 (178.5, -241.5) -> (163.5, -241.5)
  line L100 (259.5, 97.5) -> (259.5, 82.5)
  line L101 (340.5, 1.5) -> (340.5, 79.5)
  line L102 (340.5, 160.5) -> (340.5, 163.5)
  line L103 (259.5, 163.5) -> (181.5, 163.5)
  line L104 (259.5, 1.5) -> (244.5, 1.5)
  line L105 (325.5, 82.5) -> (325.5, 97.5)
  circle A15 centre (252, 90) radius 1.5
  line L106 (262.5, 241.5) -> (340.5, 241.5) construction
  circle A16 centre (333, 90) radius 1.5
  line L107 (-340.5, 1.5) -> (340.5, 1.5) construction
  line L108 (181.5, 241.5) -> (259.5, 241.5) construction
  line L109 (259.5, 16.5) -> (259.5, 1.5)
  line L110 (340.5, 241.5) -> (340.5, 163.5) construction
  line L111 (325.5, 16.5) -> (340.5, 16.5)
  line L112 (244.5, 97.5) -> (259.5, 97.5)
  line L113 (340.5, 1.5) -> (325.5, 1.5)
  line L114 (262.5, 163.5) -> (262.5, 241.5) construction
  line L115 (325.5, 97.5) -> (340.5, 97.5)
  line L116 (340.5, 16.5) -> (340.5, 1.5)
  circle A17 centre (333, 9) radius 1.5
  line L117 (259.5, 241.5) -> (262.5, 241.5) construction
  line L118 (244.5, 1.5) -> (244.5, 16.5)
  line L119 (-340.5, -82.5) -> (-340.5, -160.5)
  line L120 (-160.5, 97.5) -> (-145.5, 97.5)
  line L121 (-145.5, 163.5) -> (-223.5, 163.5)
  line L122 (-64.5, 241.5) -> (-61.5, 241.5) construction
  line L123 (340.5, -160.5) -> (340.5, -82.5)
  circle A18 centre (9, 90) radius 1.5
  line L124 (16.5, 241.5) -> (19.5, 241.5) construction
  line L125 (-160.5, -145.5) -> (-145.5, -145.5)
  line L126 (-340.5, -1.5) -> (-340.5, -79.5)
  line L127 (16.5, 241.5) -> (16.5, 163.5) construction
  line L128 (-223.5, 241.5) -> (-145.5, 241.5) construction
  circle A19 centre (9, 9) radius 1.5
  line L129 (1.5, -160.5) -> (1.5, -145.5)
  line L130 (-340.5, 163.5) -> (-340.5, 160.5)
  line L131 (-160.5, -160.5) -> (-160.5, -145.5)
  line L132 (-79.5, 1.5) -> (-79.5, 16.5)
  line L133 (-223.5, -241.5) -> (-226.5, -241.5)
  line L134 (-145.5, -79.5) -> (-160.5, -79.5)
  line L135 (1.5, 1.5) -> (1.5, 16.5)
  line L136 (-340.5, 1.5) -> (-340.5, -1.5)
  line L137 (-145.5, -241.5) -> (-160.5, -241.5)
  line L138 (-79.5, -160.5) -> (-79.5, -145.5)
  line L139 (-64.5, 1.5) -> (-79.5, 1.5)
  line L140 (-340.5, -160.5) -> (-340.5, -163.5)
  line L141 (1.5, -79.5) -> (1.5, -64.5)
  line L142 (-79.5, 82.5) -> (-79.5, 97.5)
  line L143 (-145.5, -160.5) -> (-160.5, -160.5)
  line L144 (-64.5, 16.5) -> (-64.5, 1.5)
  line L145 (1.5, 16.5) -> (16.5, 16.5)
  line L146 (-61.5, 163.5) -> (-61.5, 241.5) construction
  circle A20 centre (-153, -234) radius 1.5
  line L147 (-142.5, -241.5) -> (-145.5, -241.5)
  circle A21 centre (-72, 9) radius 1.5
  line L148 (259.5, -64.5) -> (259.5, -79.5)
  line L149 (325.5, -64.5) -> (340.5, -64.5)
  line L150 (-160.5, -241.5) -> (-160.5, -226.5)
  line L151 (-79.5, -226.5) -> (-64.5, -226.5)
  line L152 (-64.5, -226.5) -> (-64.5, -241.5)
  line L153 (-160.5, 16.5) -> (-145.5, 16.5)
  circle A22 centre (-72, -234) radius 1.5
  line L154 (-145.5, -226.5) -> (-145.5, -241.5)
  line L155 (-64.5, 241.5) -> (-64.5, 163.5) construction
  line L156 (-160.5, -79.5) -> (-160.5, -64.5)
  line L157 (1.5, 97.5) -> (16.5, 97.5)
  line L158 (1.5, -145.5) -> (16.5, -145.5)
  line L159 (-145.5, 241.5) -> (-142.5, 241.5) construction
  line L160 (-160.5, -226.5) -> (-145.5, -226.5)
  line L161 (16.5, 82.5) -> (1.5, 82.5)
  line L162 (-145.5, -145.5) -> (-145.5, -160.5)
  line L163 (-64.5, -79.5) -> (-79.5, -79.5)
  line L164 (-145.5, 82.5) -> (-160.5, 82.5)
  circle A23 centre (-153, -72) radius 1.5
  circle A24 centre (-153, -153) radius 1.5
  line L165 (-64.5, 163.5) -> (-142.5, 163.5)
  line L166 (1.5, -241.5) -> (1.5, -226.5)
  line L167 (-64.5, 97.5) -> (-64.5, 82.5)
  line L168 (-226.5, -241.5) -> (-340.5, -241.5) construction
  circle A25 centre (9, -72) radius 1.5
  line L169 (-340.5, 79.5) -> (-340.5, 1.5)
  line L170 (16.5, 97.5) -> (16.5, 82.5)
  line L171 (-145.5, 97.5) -> (-145.5, 82.5)
  line L172 (16.5, -241.5) -> (1.5, -241.5)
  circle A26 centre (-72, 90) radius 1.5
  line L173 (16.5, -160.5) -> (1.5, -160.5)
  line L174 (-340.5, -79.5) -> (-340.5, -82.5)
  line L175 (16.5, 163.5) -> (-61.5, 163.5)
  line L176 (-145.5, 241.5) -> (-145.5, 163.5) construction
  line L177 (-340.5, 82.5) -> (-340.5, 79.5)
  line L178 (1.5, -64.5) -> (16.5, -64.5)
  circle A27 centre (9, -153) radius 1.5
  line L179 (-223.5, 163.5) -> (-223.5, 241.5) construction
  circle A28 centre (-72, -72) radius 1.5
  line L180 (-340.5, 241.5) -> (-226.5, 241.5) construction
  line L181 (-64.5, -241.5) -> (-79.5, -241.5)
  line L182 (-160.5, -64.5) -> (-145.5, -64.5)
  line L183 (-64.5, -145.5) -> (-64.5, -160.5)
  line L184 (-79.5, -145.5) -> (-64.5, -145.5)
  circle A29 centre (-72, -153) radius 1.5
  line L185 (-226.5, 241.5) -> (-223.5, 241.5) construction
  line L186 (-79.5, 97.5) -> (-64.5, 97.5)
  line L187 (16.5, -79.5) -> (1.5, -79.5)
  line L188 (19.5, -241.5) -> (16.5, -241.5)
  line L189 (-340.5, 160.5) -> (-340.5, 82.5)
  line L190 (-160.5, 82.5) -> (-160.5, 97.5)
  line L191 (-142.5, 163.5) -> (-142.5, 241.5) construction
  line L192 (-64.5, -64.5) -> (-64.5, -79.5)
  line L193 (16.5, 1.5) -> (1.5, 1.5)
  line L194 (-145.5, 16.5) -> (-145.5, 1.5)
  line L195 (-79.5, -64.5) -> (-64.5, -64.5)
  line L196 (16.5, -145.5) -> (16.5, -160.5)
  line L197 (-64.5, -160.5) -> (-79.5, -160.5)
  line L198 (-79.5, -241.5) -> (-79.5, -226.5)
  line L199 (-145.5, 1.5) -> (-160.5, 1.5)
  circle A30 centre (-153, 90) radius 1.5
  line L200 (-160.5, 1.5) -> (-160.5, 16.5)
  line L201 (1.5, -226.5) -> (16.5, -226.5)
  line L202 (-145.5, -64.5) -> (-145.5, -79.5)
  line L203 (-79.5, -79.5) -> (-79.5, -64.5)
  line L204 (16.5, -64.5) -> (16.5, -79.5)
  line L205 (-61.5, -241.5) -> (-64.5, -241.5)
  circle A31 centre (-153, 9) radius 1.5
  circle A32 centre (9, -234) radius 1.5
  line L206 (-340.5, -79.5) -> (340.5, -79.5) construction
  line L207 (259.5, -241.5) -> (259.5, 241.5) construction
  line L208 (-340.5, 160.5) -> (340.5, 160.5) construction
  line L209 (340.5, 82.5) -> (-340.5, 82.5) construction
  line L210 (-340.5, -241.5) -> (-340.5, 241.5) construction
  line L211 (181.5, 241.5) -> (181.5, -241.5) construction
  circle A33 centre (171, -72) radius 1.5
  line L212 (262.5, 241.5) -> (262.5, -241.5) construction
  line L213 (340.5, -79.5) -> (-340.5, -79.5) construction
  line L214 (82.5, -160.5) -> (82.5, -145.5)
  line L215 (340.5, -82.5) -> (-340.5, -82.5) construction
  line L216 (-145.5, -241.5) -> (-145.5, 241.5) construction
  line L217 (340.5, 160.5) -> (-340.5, 160.5) construction
  line L218 (340.5, 1.5) -> (-340.5, 1.5) construction
  line L219 (340.5, -241.5) -> (340.5, 241.5) construction
  line L220 (325.5, -226.5) -> (340.5, -226.5)
  line L221 (325.5, -79.5) -> (325.5, -64.5)
  line L222 (259.5, -160.5) -> (244.5, -160.5)
  line L223 (-340.5, -241.5) -> (340.5, -241.5) construction
  line L224 (340.5, -226.5) -> (340.5, -241.5)
  line L225 (-226.5, -241.5) -> (-226.5, 241.5) construction
  circle A34 centre (333, -234) radius 1.5
  line L226 (-340.5, 79.5) -> (340.5, 79.5) construction
  line L227 (82.5, -226.5) -> (97.5, -226.5)
  line L228 (100.5, 241.5) -> (100.5, -241.5) construction
  line L229 (97.5, -241.5) -> (97.5, 241.5) construction
  line L230 (19.5, 241.5) -> (19.5, -241.5) construction
  line L231 (-340.5, -160.5) -> (340.5, -160.5) construction
  line L232 (340.5, -160.5) -> (-340.5, -160.5) construction
  line L233 (-142.5, 241.5) -> (-142.5, -241.5) construction
  line L234 (244.5, -79.5) -> (244.5, -64.5)
  line L235 (-64.5, -241.5) -> (-64.5, 241.5) construction
  line L236 (259.5, -145.5) -> (259.5, -160.5)
  line L237 (178.5, -241.5) -> (178.5, 241.5) construction
  line L238 (-61.5, 241.5) -> (-61.5, -241.5) construction
  line L239 (-172.5, -238.5) -> (-172.5, -228.5)
  circle A35 centre (-153, -228.4307) radius 1.5
  line L240 (-172.5, -228.5) -> (-154.5, -228.436)
  circle A36 centre (-72, -228.1428) radius 1.5
  line L241 (-151.5, -228.4254) -> (-73.5, -228.1481)
  circle A37 centre (9, -227.8549) radius 1.5
  line L242 (-70.5, -228.1375) -> (7.5, -227.8602)
  circle A38 centre (90, -227.567) radius 1.5
  line L243 (10.5, -227.8495) -> (88.5, -227.5723)
  circle A39 centre (171, -227.2791) radius 1.5
  circle A40 centre (252, -226.9912) radius 1.5
  line L244 (244.5, -226.5) -> (250.5827, -226.5)
  line L245 (253.4173, -226.5) -> (259.5, -226.5)
  line L246 (91.5, -227.5616) -> (250.5, -226.9965)
  line L247 (253.5, -226.9858) -> (390.1836, -226.5)
  point P0 (-172.5, -238.5)
  dimension "d102" = 114
  dimension "d103" = 3
  dimension "d104" = 78
  dimension "d105" = 78
  dimension "d15" = 3
  dimension "d16" = 78
  dimension "d108" = 78
  dimension "d109" = 3
  dimension "d110" = 78
  dimension "d111" = 78
  dimension "d112" = 3
  dimension "d113" = 78
  dimension "d114" = 78
  dimension "d115" = 3
  dimension "d116" = 78
  dimension "d117" = 78
  dimension "d118" = 3
  dimension "d119" = 78
  dimension "d120" = 78
  dimension "d121" = 3
  dimension "d122" = 483
  dimension "d32" = 78
  dimension "d33" = 3
  dimension "d34" = 78
  dimension "d35" = 3
  dimension "d36" = 78
  dimension "d37" = 3
  dimension "d38" = 78
  dimension "d39" = 3
  dimension "d40" = 78
  dimension "d41" = 3
  dimension "d42" = 15
  dimension "d43" = 15
  dimension "d44" = 15
  dimension "d45" = 15
  dimension "d46" = 15
  dimension "d47" = 15
  dimension "d48" = 15
  dimension "d49" = 15
  dimension "d50" = 15
  dimension "d51" = 15
  dimension "d52" = 15
  dimension "d53" = 15
  dimension "d54" = 15
  dimension "d55" = 15
  dimension "d56" = 15
  dimension "d57" = 15
  dimension "d58" = 15
  dimension "d59" = 15
  dimension "d60" = 15
  dimension "d61" = 15
  dimension "d62" = 15
  dimension "d63" = 15
  dimension "d64" = 15
  dimension "d65" = 15
  dimension "d66" = 15
  dimension "d67" = 15
  dimension "d68" = 15
  dimension "d69" = 15
  dimension "d70" = 15
  dimension "d71" = 15
  dimension "d72" = 15
  dimension "d73" = 15
  dimension "d74" = 15
  dimension "d75" = 15
  dimension "d76" = 15
  dimension "d77" = 15
  dimension "d78" = 15
  dimension "d79" = 15
  dimension "d80" = 15
  dimension "d81" = 15
  dimension "d82" = 15
  dimension "d83" = 15
  dimension "d84" = 15
  dimension "d85" = 15
  dimension "d86" = 15
  dimension "d87" = 15
  dimension "d88" = 15
  dimension "d89" = 15
  dimension "d90" = 15
  dimension "d91" = 15
  dimension "d92" = 15
  dimension "d93" = 15
  dimension "d94" = 15
  dimension "d95" = 15
  dimension "d96" = 15
  dimension "d97" = 15
  dimension "d98" = 15
  dimension "d99" = 15
  dimension "d100" = 15
  dimension "d101" = 15
  dimension "d193" = 15
  dimension "d194" = 15
  dimension "d195" = 15
  dimension "d196" = 15
  dimension "d106" = 15
  dimension "d107" = 15
  dimension "d199" = 15
  dimension "d200" = 15
  dimension "d201" = 15
  dimension "d202" = 15
  dimension "d203" = 3
  dimension "d204" = 3
  dimension "d205" = 3
  dimension "d206" = 3
  dimension "d207" = 3
  dimension "d208" = 3
  dimension "d209" = 3
  dimension "d210" = 3
  dimension "d211" = 3
  dimension "d212" = 3
  dimension "d213" = 3
  dimension "d123" = 3
  dimension "d124" = 3
  dimension "d125" = 3
  dimension "d126" = 3
  dimension "d127" = 3
  dimension "d128" = 3
  dimension "d129" = 3
  dimension "d130" = 3
  dimension "d131" = 3
  dimension "d132" = 3
  dimension "d133" = 3
  dimension "d134" = 3
  dimension "d135" = 3
  dimension "d136" = 3
  dimension "d137" = 3
  dimension "d138" = 3
  dimension "d139" = 3
  dimension "d140" = 3
  dimension "d141" = 3
  dimension "d142" = 3
  dimension "d143" = 3
  dimension "d144" = 3
  dimension "d145" = 3
  dimension "d146" = 3
  dimension "d149" = 151.5
  dimension "d150" = 81
  dimension "d151" = 81
  dimension "d152" = 81
  dimension "d153" = 81
  dimension "d154" = 7.5
  dimension "d155" = 187.5
  dimension "d156" = 81
  dimension "d157" = 81
  dimension "d158" = 81
  dimension "d159" = 81
  dimension "d160" = 81
  dimension "d161" = 81
  dimension "d251" = 10
  dimension "d252" = 3
  dimension "d253" = 3
  dimension "d254" = 3
  dimension "d255" = 3
  dimension "d256" = 3
  dimension "d257" = 3
  constraint horizontal L180
  constraint vertical L80
  constraint horizontal L168
  constraint vertical L210
  constraint coincident L51.end L89.start
  constraint horizontal L185
  constraint vertical L76
  constraint horizontal L133
  constraint vertical L225
  constraint horizontal L128
  constraint vertical L176
  constraint horizontal L121
  constraint vertical L179
  constraint horizontal L159
  constraint vertical L233
  constraint horizontal L147
  constraint vertical L216
  constraint horizontal L78
  constraint vertical L155
  constraint horizontal L165
  constraint vertical L191
  constraint horizontal L122
  constraint vertical L238
  constraint horizontal L205
  constraint vertical L235
  constraint horizontal L79
  constraint vertical L127
  constraint horizontal L175
  constraint vertical L146
  constraint horizontal L124
  constraint vertical L230
  constraint horizontal L188
  constraint vertical L85
  constraint horizontal L9
  constraint vertical L5
  constraint horizontal L28
  constraint vertical L69
  constraint horizontal L10
  constraint vertical L228
  constraint horizontal L98
  constraint vertical L229
  constraint horizontal L22
  constraint vertical L16
  constraint horizontal L3
  constraint vertical L25
  constraint horizontal L2
  constraint vertical L211
  constraint horizontal L96
  constraint vertical L237
  constraint horizontal L108
  constraint vertical L15
  constraint horizontal L103
  constraint vertical L6
  constraint horizontal L117
  constraint vertical L212
  constraint horizontal L86
  constraint vertical L207
  constraint horizontal L106
  constraint vertical L110
  constraint horizontal L24
  constraint vertical L114
  constraint horizontal L43
  constraint vertical L130
  constraint horizontal L208
  constraint vertical L102
  constraint horizontal L217
  constraint vertical L189
  constraint horizontal L42
  constraint vertical L14
  constraint horizontal L209
  constraint vertical L177
  constraint horizontal L226
  constraint vertical L23
  constraint horizontal L38
  constraint vertical L169
  constraint horizontal L107
  constraint vertical L101
  constraint horizontal L218
  constraint vertical L136
  constraint horizontal L48
  constraint vertical L54
  constraint horizontal L11
  constraint vertical L126
  constraint horizontal L206
  constraint vertical L61
  constraint horizontal L213
  constraint vertical L174
  constraint horizontal L8
  constraint vertical L83
  constraint horizontal L215
  constraint vertical L119
  constraint horizontal L231
  constraint vertical L123
  constraint horizontal L232
  constraint vertical L140
  constraint horizontal L40
  constraint vertical L74
  constraint horizontal L164
  constraint vertical L190
  constraint horizontal L120
  constraint vertical L171
  constraint coincident L164.start L216
  constraint coincident L164.start L42
  constraint horizontal L82
  constraint vertical L142
  constraint horizontal L186
  constraint vertical L167
  constraint coincident L82.start L235
  constraint coincident L82.start L209
  constraint horizontal L161
  constraint vertical L84
  constraint horizontal L157
  constraint vertical L170
  constraint coincident L161.start L42
  constraint coincident L161.start L85
  constraint horizontal L199
  constraint vertical L200
  constraint horizontal L153
  constraint vertical L194
  constraint coincident L194.end L216
  constraint coincident L194.end L218
  constraint horizontal L139
  constraint vertical L132
  constraint horizontal L87
  constraint vertical L144
  constraint coincident L139.start L235
  constraint coincident L139.start L218
  constraint horizontal L193
  constraint vertical L135
  constraint horizontal L145
  constraint vertical L63
  constraint coincident L63.end L85
  constraint coincident L63.end L107
  constraint horizontal L134
  constraint vertical L156
  constraint horizontal L182
  constraint vertical L202
  constraint coincident L134.start L216
  constraint coincident L134.start L206
  constraint horizontal L143
  constraint vertical L131
  constraint horizontal L125
  constraint vertical L162
  constraint coincident L143.start L216
  constraint coincident L143.start L231
  constraint horizontal L163
  constraint vertical L203
  constraint horizontal L195
  constraint vertical L192
  constraint coincident L163.start L235
  constraint coincident L163.start L213
  constraint horizontal L197
  constraint vertical L138
  constraint horizontal L184
  constraint vertical L183
  constraint coincident L183.end L235
  constraint coincident L183.end L231
  constraint horizontal L173
  constraint vertical L129
  constraint horizontal L158
  constraint vertical L196
  constraint coincident L173.start L231
  constraint coincident L173.start L85
  constraint horizontal L187
  constraint vertical L141
  constraint horizontal L178
  constraint vertical L204
  constraint coincident L187.start L206
  constraint coincident L187.start L85
  constraint horizontal L137
  constraint vertical L150
  constraint horizontal L160
  constraint vertical L154
  constraint horizontal L181
  constraint vertical L198
  constraint horizontal L151
  constraint vertical L152
  constraint horizontal L172
  constraint vertical L166
  constraint horizontal L201
  constraint vertical L62
  constraint horizontal L7
  constraint vertical L12
  constraint horizontal L20
  constraint vertical L13
  constraint coincident L7.start L229
  constraint coincident L7.start L209
  constraint horizontal L4
  constraint vertical L31
  constraint horizontal L29
  constraint vertical L30
  constraint coincident L4.start L237
  constraint coincident L4.start L42
  constraint horizontal L57
  constraint vertical L17
  constraint horizontal L112
  constraint vertical L100
  constraint coincident L57.start L207
  constraint coincident L57.start L209
  constraint horizontal L32
  constraint vertical L0
  constraint horizontal L27
  constraint vertical L21
  constraint coincident L21.end L229
  constraint coincident L21.end L107
  constraint horizontal L33
  constraint vertical L34
  constraint horizontal L1
  constraint vertical L26
  constraint coincident L26.end L237
  constraint coincident L26.end L218
  constraint horizontal L36
  constraint vertical L39
  constraint horizontal L50
  constraint vertical L44
  constraint coincident L36.start L229
  constraint coincident L36.start L206
  constraint horizontal L94
  constraint vertical L52
  constraint horizontal L35
  constraint vertical L90
  constraint coincident L90.end L237
  constraint coincident L90.end L206
  constraint horizontal L56
  constraint vertical L214
  constraint horizontal L91
  constraint vertical L92
  constraint coincident L56.start L229
  constraint coincident L56.start L232
  constraint horizontal L95